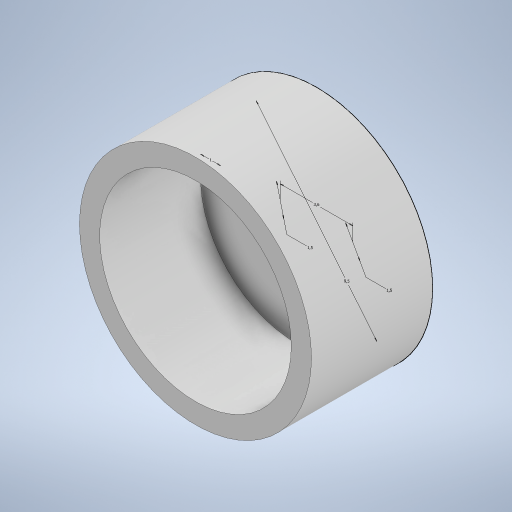
# Autodesk Inventor part: El_Cap_Support
Saved by Autodesk Inventor 2024 (Build 280153000, 153)
## iProperties
Created: 2026-06-13
Part Number: El_Cap_Support
Material: Типовые
Document SubType Name: Modeling
Designer: fm
Density: 1 g/cm^3
Appearance: По умолчанию
Author: fm
Autodesk Inventor part; units mm, degrees
ref_plane "YZ Plane" through (0, 0, 0) normal (1, 0, 0) x (0, 1, 0)
ref_plane "XZ Plane" through (0, 0, 0) normal (0, 1, 0) x (-1, 0, 0)
ref_plane "XY Plane" through (0, 0, 0) normal (0, 0, 1) x (1, 0, 0)
sketch "Эскиз1" plane through (0, 0, 0) normal (0, 0, 1) x (1, 0, 0)
  circle A0 centre (0, 0) radius 4.75
  line L0 (-1.8, 0) -> (1.8, 0) construction
  circle A1 centre (-1.8, 0) radius 0.75
  circle A2 centre (1.8, 0) radius 0.75
  circle A3 centre (0, 0) radius 5.75
  dimension "d0" = 9.5
  dimension "d1" = 3.6
  dimension "d2" = 1.5
  dimension "d3" = 1.5
  dimension "d4" = 1
  constraints: 4 centre point, 4 coincident, 2 end point, 1 horizontal, 1 midpoint
  measures "d0" diameter of A0
  measures "d1" distance of L0.start L0.end
  measures "d2" diameter of A1
  measures "d3" diameter of A2
  measures "d4" radial gap between concentric circles of A0 A3
extrude "Выдавливание1" add sketch "Эскиз1" along normal blind 1 contours A0 | A3
extrude "Выдавливание2" add sketch "Эскиз1" along normal blind 5 from surface at 1 contours A3
